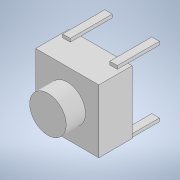
# Autodesk Inventor part: Button
Saved by Autodesk Inventor 2022 (Build 260153000, 153)
## iProperties
Created: 2022-10-09
Part Number: Button
Material: Generic
Document SubType Name: Modeling
Designer: Nick
Density: 1 g/cm^3
Appearance: Default
Author: Nick
Autodesk Inventor part; units mm, degrees
ref_plane "YZ Plane" through (0, 0, 0) normal (1, 0, 0) x (0, 1, 0)
ref_plane "XZ Plane" through (0, 0, 0) normal (0, 1, 0) x (-1, 0, 0)
ref_plane "XY Plane" through (0, 0, 0) normal (0, 0, 1) x (1, 0, 0)
sketch "Sketch1" plane through (0, 0, 0) normal (0, 0, 1) x (1, 0, 0)
  line L0 (0, 0) -> (6, 0)
  line L1 (6, 0) -> (6, 6)
  line L2 (6, 6) -> (0, 6)
  line L3 (0, 6) -> (0, 0)
  dimension "d0" = 6
  dimension "d1" = 6
  constraints: 8 end point, 2 parallel, 1 horizontal, 1 perpendicular
  measures "d0" distance of L2.end L1.end
  measures "d1" distance of L1.end L0.end
extrude "Extrusion1" add sketch "Sketch1" along normal blind 3.16
sketch "Sketch2" plane through (0, 0, 3.16) normal (0, 0, 1) x (1, 0, 0)
  circle A0 centre (3, 3) radius 1.735
  line L0 (6, 0) -> (6, 6) projected
  line L1 (6, 6) -> (0, 6) projected
  point P0 (0, 0)
  point P1 (6, 3)
  point P2 (3, 6)
  dimension "d4" = 3.47
  constraints: 2 midpoint, 1 centre point, 1 horizontal alignment, 1 vertical alignment
  measures "d4" diameter of A0
extrude "Extrusion2" add sketch "Sketch2" along normal blind 1.84
sketch "Sketch3" plane through (0, 0, 0) normal (0, 0, -1) x (-1, 0, 0)
  line L0 (-5.6, 6.31) -> (-4.88, 6.31)
  line L1 (-4.88, 6.31) -> (-4.88, 6)
  line L2 (-4.88, 6) -> (-5.6, 6)
  line L3 (-5.6, 6) -> (-5.6, 6.31)
  line L4 (-6, 6) -> (0, 6) projected
  line L5 (-6, 0) -> (-6, 6) projected
  point P0 (0, 0)
  dimension "d7" = 0.72
  dimension "d8" = 0.31
  dimension "d9" = 0.4
  constraints: 8 end point, 2 parallel, 1 collinear, 1 horizontal, 1 perpendicular
  measures "d7" distance of L0.start L0.end
  measures "d8" distance of L2.end L0.start
  measures "d9" distance between parallel lines of L5 L3
extrude "Extrusion3" add sketch "Sketch3" along normal blind 3 and the other way blind 1
ref_plane "Work Plane1" through (3, 0, 0) normal (1, 0, 0) x (0, 0, -1)
ref_plane "Work Plane2" through (0, 3, 0) normal (0, -1, 0) x (1, 0, 0)
mirror "Mirror3" about plane through (3, 0, 0) normal (1, 0, 0) of "Extrusion3"
mirror "Mirror4" about plane through (0, 3, 0) normal (0, -1, 0) of "Extrusion3", "Mirror3"
body "Solid1"
